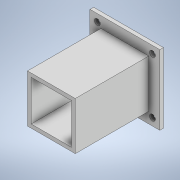
# Autodesk Inventor part: pmtholder
Saved by Autodesk Inventor 2022.2 (Build 262287030, 287C)
## iProperties
Created: 2022-03-11
Part Number: pmtholder
Material: Generic
Document SubType Name: Modeling
Designer: Tapendra
Density: 1 g/cm^3
Appearance: Default
Author: Tapendra
Autodesk Inventor part; units mm, degrees
ref_plane "YZ Plane" through (0, 0, 0) normal (1, 0, 0) x (0, 1, 0)
ref_plane "XZ Plane" through (0, 0, 0) normal (0, 1, 0) x (-1, 0, 0)
ref_plane "XY Plane" through (0, 0, 0) normal (0, 0, 1) x (1, 0, 0)
sketch "Sketch1" plane through (0, 0, 0) normal (0, 0, 1) x (1, 0, 0)
  line L0 (-19, 19) -> (19, 19)
  line L1 (19, 19) -> (19, -19)
  line L2 (19, -19) -> (-19, -19)
  line L3 (-19, -19) -> (-19, 19)
  line L4 (-19, 19) -> (19, -19) construction
  line L5 (19, 19) -> (-19, -19) construction
  line L6 (-11, 11) -> (11, 11)
  line L7 (11, 11) -> (11, -11)
  line L8 (11, -11) -> (-11, -11)
  line L9 (-11, -11) -> (-11, 11)
  line L10 (-11, 11) -> (11, -11) construction
  line L11 (11, 11) -> (-11, -11) construction
  point P0 (0, 0)
  dimension "d0" = 38
  dimension "d1" = 38
  dimension "d2" = 22
  dimension "d3" = 22
  constraints: 24 end point, 4 midpoint, 4 parallel, 2 horizontal, 2 perpendicular
  measures "d0" distance of L0.end L1.end
  measures "d1" distance of L0.start L0.end
  measures "d2" distance of L6.end L7.end
  measures "d3" distance of L6.start L6.end
extrude "Extrusion1" add sketch "Sketch1" along normal mid plane 2
sketch "Sketch2" plane through (0, 0, 1) normal (0, 0, 1) x (1, 0, 0)
  line L0 (-13, 13) -> (13, 13)
  line L1 (13, 13) -> (13, -13)
  line L2 (13, -13) -> (-13, -13)
  line L3 (-13, -13) -> (-13, 13)
  line L4 (-13, 13) -> (13, -13) construction
  line L5 (13, 13) -> (-13, -13) construction
  line L6 (-11, -11) -> (11, -11)
  line L7 (11, -11) -> (11, 11)
  line L8 (11, 11) -> (-11, 11)
  line L9 (-11, 11) -> (-11, -11)
  line L10 (-11, -11) -> (11, 11) construction
  line L11 (11, -11) -> (-11, 11) construction
  point P0 (0, 0)
  dimension "d6" = 26
  dimension "d7" = 26
  dimension "d8" = 22
  constraints: 24 end point, 4 midpoint, 4 parallel, 2 horizontal, 2 perpendicular, 1 point on line
  measures "d6" distance of L0.end L1.end
  measures "d7" distance of L0.start L0.end
  measures "d8" distance of L6.end L7.end
extrude "Extrusion2" add sketch "Sketch2" along normal blind 40
sketch "Sketch3" plane through (0, 0, -1) normal (0, 0, -1) x (-1, 0, 0)
  line L0 (11, -11) -> (11, 11) projected
  line L1 (11, 11) -> (-11, 11) projected
  line L2 (-11, 11) -> (-11, -11) projected
  line L3 (-11, -11) -> (11, -11) projected
  line L4 (19, 19) -> (19, -19) projected
  line L5 (19, -19) -> (-19, -19) projected
  line L6 (-19, -19) -> (-19, 19) projected
  line L7 (-19, 19) -> (19, 19) projected
  point P0 (0, 0)
  point P1 (15, -15)
  point P2 (-15, -15)
  point P3 (15, 15)
  point P4 (-15, 15)
  dimension "d11" = 15
  dimension "d12" = 15
  dimension "d15" = 30
  dimension "d18" = 30
  constraints: 1 horizontal, 1 vertical, 3 other
  measures "d11" horizontal distance of point (15, -15) point (0, 0)
  measures "d12" horizontal distance of point (15, -15) point (0, 0)
  measures "d15" distance of point (15, -15) point (-15, -15)
  measures "d18" distance of point (15, -15) point (15, 15)
hole "Hole1" at (-15, -15, -1) at (15, -15, -1) at (-15, 15, -1) at (15, 15, -1) direction (0, 0, 1) diameter 3.242 end through all thread size "M4x0.7" class "6H" standard "ANSI Metric M Profile"
equation "\"d1\" = d0"
equation "\"d3\" = d2"
equation "\"d7\" = d6"
body "Solid1"
